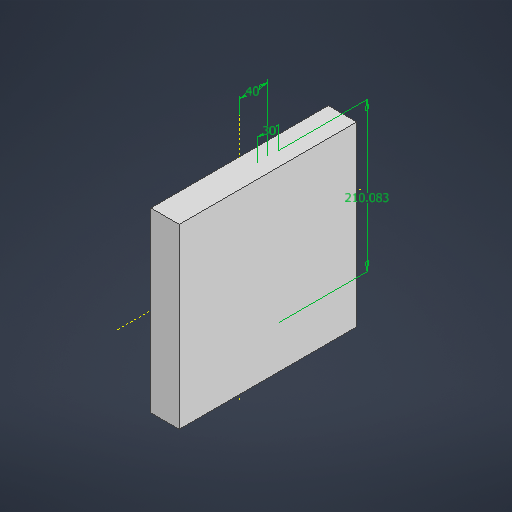
# Autodesk Inventor part: Suspension_Upright_V2_Topology_Baseline_V1
Saved by Autodesk Inventor 2026.1 (Build 301233000, 233)
## iProperties
Created: 2026-09-05
Part Number: Suspension_Upright_V2_Topology_Baseline_V1
Material: Generic
Document SubType Name: Modeling
Designer: share
Density: 1 g/cm^3
Appearance: Default
Author: share
Autodesk Inventor part; units mm, degrees
ref_plane "YZ Plane" through (0, 0, 0) normal (1, 0, 0) x (0, 1, 0)
ref_plane "XZ Plane" through (0, 0, 0) normal (0, 1, 0) x (-1, 0, 0)
ref_plane "XY Plane" through (0, 0, 0) normal (0, 0, 1) x (1, 0, 0)
sketch "Sketch1" plane through (0, 0, 0) normal (1, 0, 0) x (0, 1, 0)
  line L0 (0, 175) -> (0, -175) construction
  line L1 (-175, 0) -> (175, 0) construction
  line L2 (125, 125) -> (-125, 125)
  line L3 (-125, 125) -> (-125, -125)
  line L4 (-125, -125) -> (125, -125)
  line L5 (125, -125) -> (125, 125)
  point P0 (0, 0)
  dimension "d0" = 250
  dimension "d1" = 250
  constraints: 8 end point, 2 parallel, 1 horizontal, 1 perpendicular, 2 other
  measures "d0" distance between parallel lines of L4 L2
  measures "d1" distance between parallel lines of L3 L5
extrude "Extrusion1" add sketch "Sketch1" along normal blind 40
sketch "Sketch4" plane through (0, 0, 0) normal (-1, 0, 0) x (0, 0, 1)
  line L0 (-175, 0) -> (175, 0) construction
  line L1 (0, 175) -> (0, -175) construction
  line L2 (-55, 105.0416) -> (-25, 105.0416) construction
  line L3 (-55, -105.0416) -> (-25, -105.0416) construction
  line L4 (-40, 105.0416) -> (-40, -105.0416) construction
  point P0 (0, 0)
  dimension "d10" = 30
  dimension "d12" = 40
  dimension "d13" = 210.0832
  constraints: 6 end point, 2 horizontal, 2 midpoint, 2 symmetric about line, 1 parallel
  measures "d10" distance of L2.end L2.start
  measures "d12" distance between parallel lines of L1 L4
  measures "d13" distance between parallel lines of L3 L2
body "Solid1"
